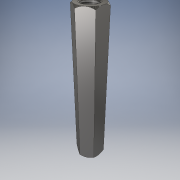
# Autodesk Inventor part: PillarBolt-M3x30
Saved by Autodesk Inventor 2018 (Build 220112000, 112)
## iProperties
Created: 2020-04-17
Part Number: PillarBolt-M3x30
Material: Ocel, vysokopevnostní, nízkolegovaná
Document SubType Name: Modeling
Designer: Jozko Mrkvicka
Density: 7.85 g/cm^3
Appearance: Ocel – leštěná
Author: Jozko Mrkvicka
Autodesk Inventor part; units mm, degrees
ref_plane "YZ Plane" through (0, 0, 0) normal (1, 0, 0) x (0, 1, 0)
ref_plane "XZ Plane" through (0, 0, 0) normal (0, 1, 0) x (-1, 0, 0)
sketch "Náčrt1" plane through (0, 0, 0) normal (0, 0, 1) x (1, 0, 0)
  line L0 (2.5, -1.4434) -> (0, -2.8868)
  line L1 (0, -2.8868) -> (-2.5, -1.4434)
  line L2 (-2.5, -1.4434) -> (-2.5, 1.4434)
  line L3 (-2.5, 1.4434) -> (0, 2.8868)
  line L4 (0, 2.8868) -> (2.5, 1.4434)
  line L5 (2.5, 1.4434) -> (2.5, -1.4434)
  circle A0 centre (0, 0) radius 1.5
  point P0 (2.5, 0)
  dimension "d1" = 3
  dimension "d16" = 5
  constraints: 12 end point, 1 centre point, 1 coincident, 1 midpoint, 13 other
  measures "d1" diameter of A0
  measures "d16" distance between parallel lines of L5 L2
extrude "Vysunutí1" add sketch "Náčrt1" along normal blind 30
thread "Závit1" size "M3x0.5" class "6H" standard "ANSI Metric M Profile" full length
sketch "Náčrt2" plane through (0, 0, 30) normal (0, 0, 1) x (1, 0, 0)
  circle A0 centre (0, 0) radius 2.5
  dimension "d18" = 5
  constraints: 1 centre point, 1 coincident
  measures "d18" diameter of A0
extrude "Vysunutí2" cut sketch "Náčrt2" against normal through all draft 45 keep common part
sketch "Náčrt3" plane through (0, 0, 0) normal (0, 0, -1) x (-1, 0, 0)
  circle A0 centre (0, 0) radius 2.5
  dimension "d17" = 5
  constraints: 1 centre point, 1 coincident
  measures "d17" diameter of A0
extrude "Vysunutí3" cut sketch "Náčrt3" against normal through all draft 45 keep common part
chamfer "Zkosení1" distance 0.2 angle 45 1 edges at (-1.5, 0, 30)
chamfer "Zkosení2" distance 0.2 angle 45 1 edges at (-1.5, 0, 0)
ref_plane "Pracovní rovina1" through (0, 0, 15) normal (0, 0, -1) x (-1, 0, 0)
sketch "Náčrt4" plane through (-2.5, 1.4434, 29.6132) normal (-0.5, 0.8660254, 0) x (0.8660254, 0.5, 0)
  point P0 (1.4434, 29.6132)
sketch "Náčrt5" plane through (0, 0, 15) normal (0, 0, -1) x (-1, 0, 0)
  circle A0 centre (0, 0) radius 1.5
  constraints: 1 centre point, 1 coincident
extrude "Vysunutí4" add sketch "Náčrt5" along normal mid plane 8
